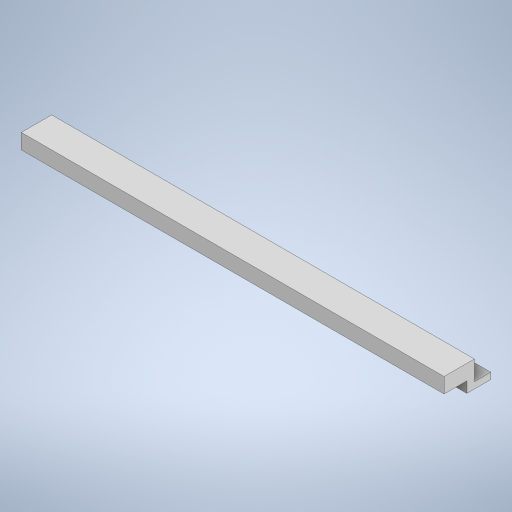
# Autodesk Inventor part: porta guide
Saved by Autodesk Inventor 2024 (Build 280153000, 153)
## iProperties
Created: 2024-03-01
Part Number: porta guide
Material: Generico
Document SubType Name: Modeling
Designer: Giorgio
Density: 1 g/cm^3
Appearance: Default
Author: Giorgio
Autodesk Inventor part; units mm, degrees
ref_plane "YZ Plane" through (0, 0, 0) normal (1, 0, 0) x (0, 1, 0)
ref_plane "XZ Plane" through (0, 0, 0) normal (0, 1, 0) x (-1, 0, 0)
ref_plane "XY Plane" through (0, 0, 0) normal (0, 0, 1) x (1, 0, 0)
sketch "Schizzo1" plane through (0, 0, 0) normal (1, 0, 0) x (0, 1, 0)
  line L0 (87.11, -30.7543) -> (73.11, -30.7543)
  line L1 (73.11, -23.7543) -> (73.11, -2.7543)
  line L2 (73.11, -2.7543) -> (87.11, -2.7543)
  line L3 (87.11, -2.7543) -> (87.11, -30.7543)
  line L4 (73.11, -30.7543) -> (69.11, -30.7543)
  line L5 (63.11, -30.7543) -> (63.11, -23.7543)
  line L6 (63.11, -23.7543) -> (73.11, -23.7543)
  line L7 (69.11, -30.7543) -> (69.11, -45.7543)
  line L8 (69.11, -45.7543) -> (63.11, -45.7543)
  line L9 (63.11, -45.7543) -> (63.11, -30.7543)
  constraints: 20 end point, 4 parallel, 2 horizontal, 2 perpendicular
extrude "Estrusione2" add sketch "Schizzo1" along normal blind 390
